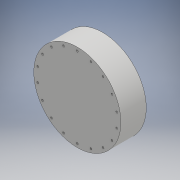
# Autodesk Inventor part: Korbbogenboden
Saved by Autodesk Inventor 2017 (Build 210142000, 142)
## iProperties
Created: 2019-06-21
Part Number: Korbbogenboden
Material: Generic
Document SubType Name: Modeling
Designer: Ole Simmering
Density: 1 g/cm^3
Appearance: Default
Author: Ole Simmering
Autodesk Inventor part; units mm, degrees
ref_plane "YZ Plane" through (0, 0, 0) normal (1, 0, 0) x (0, 1, 0)
ref_plane "XY Plane" through (0, 0, 0) normal (0, 0, 1) x (1, 0, 0)
sketch "Sketch1" plane through (0, 0, 0) normal (0, 0, 1) x (1, 0, 0)
  line L0 (0, -110.6871) -> (0, 217.0976)
  line L1 (144, 0) -> (144, -18)
  arc A0 (121.1146, -57.8857) -> (144, -18) centre (97.8, -18) ccw
  arc A1 (0, -90.6871) -> (121.1146, -57.8857) centre (0, 149.3129) ccw
  line L2 (144, 0) -> (190, 0)
  line L3 (144, -18) -> (97.8, -18) construction
  line L4 (121.1146, -57.8857) -> (97.8, -18) construction
  line L5 (0, -90.6871) -> (0, -110.6871) construction
  line L6 (0, -110.6871) -> (190, -110.6871)
  line L7 (190, -110.6871) -> (190, 0)
  line L8 (0, -90.6871) -> (0, -110.6871)
  line L9 (144, 0) -> (190, 0)
  point P0 (0, 0)
  dimension "d0" = 288
  dimension "d19" = 380
  dimension "d20" = 20
  dimension "d22" = 18
  dimension "d23" = 46.2
  dimension "d24" = 240
  dimension "d26" = 46
  constraints: 21 end point, 4 point on circle, 4 point on line, 3 horizontal, 2 centre point, 2 collinear, 2 tangent, 2 vertical, 1 line through centre, 1 perpendicular
  measures "d0" diameter of L1 L0
  measures "d19" diameter of L7 L0
  measures "d20" distance of L5.start L0.start
  measures "d22" distance of L1.start L1.end
  measures "d23" radius of A0
  measures "d24" radius of A1
  measures "d26" distance of L1.start L9.end
revolve "Revolution1" add sketch "Sketch1" angle 360 about axis through (0, -110.6871, 0) along (0, 1, 0)
ref_plane "Work Plane1" through (0, -100, 0) normal (0, 1, 0) x (-1, 0, 0)
sketch "Sketch2" plane through (0, -110.6871, 0) normal (0, -1, 0) x (1, 0, 0)
  circle A0 centre (0, 0) radius 190 construction
  point P0 (0, 0)
  point P1 (0, -175)
  point P2 (0, 0)
  dimension "d8" = 175
  constraints: 1 centre point, 1 coincident
  measures "d8" distance of point (0, 0) point (0, -175)
hole "Hole1" at (0, -110.6871, -175) direction (0, 1, 0) diameter 8.376 end through all thread size "M10x1.5" class "6H" standard "ISO Metric profile"
pattern_circular "Circular Pattern1" count 18 over 360 about axis through (0, -9, 0) along (0, 1, 0) of "Hole1"
body "Solid1"
